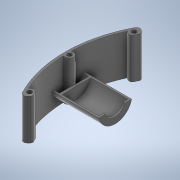
# Autodesk Inventor part: side_prot_cap
Saved by Autodesk Inventor 2020 (Build 240168000, 168)
## iProperties
Created: 2023-12-20
Part Number: side_prot_cap
Material: Пластик АБС
Document SubType Name: Modeling
Designer: denis
Density: 1.06 g/cm^3
Appearance: Гладкая — черная
Author: denis
## iProperties of the stored document _3DПЕЧАТЬ.ipt
Created: 2024-05-20
Part Number: _3DПЕЧАТЬ
Material: Типовые
Document SubType Name: Modeling
Designer: 4s
Density: 1 g/cm^3
Appearance: По умолчанию
Author: 4s
Autodesk Inventor part; units mm, degrees
(part 1 of 3)
ref_plane "XZ Plane" through (0, 0, 0) normal (0, 1, 0) x (-1, 0, 0)
sketch "Эскиз1" plane through (0, 0, 0) normal (0, 1, 0) x (-1, 0, 0)
  arc A0 (93.0503, -48.6481) -> (93.0503, 48.6481) centre (0, 0) ccw
  line L0 (0, 0) -> (0, -105) construction
  line L1 (0, 0) -> (105, 0) construction
  line L2 (0, 0) -> (74.2462, -74.2462) construction
  line L3 (0, 0) -> (105, 0) construction
  arc A1 (47.0668, -85.9577) -> (85.9577, -47.0668) centre (0, 0) ccw construction
  line L4 (0, 0) -> (-74.2462, -74.2462) construction
  line L5 (73.8927, -46.3155) -> (46.3155, -73.8927)
  line L6 (76.014, -34.2947) -> (34.2947, -76.014)
  circle A2 centre (37.8302, -79.5495) radius 1.6
  circle A3 centre (79.5495, -37.8302) radius 1.6
  line L7 (37.8302, -79.5495) -> (79.5495, -37.8302) construction
  line L8 (87.1795, -38.3892) -> (83.085, -34.2947)
  line L9 (38.3892, -87.1795) -> (34.2947, -83.085)
  line L10 (88.2704, -49.3795) -> (85.2064, -46.3155)
  line L11 (49.3795, -88.2704) -> (46.3155, -85.2064)
  arc A4 (74.2462, -74.2462) -> (91.1, -52.2091) centre (0, 0) ccw construction
  arc A5 (52.2091, -91.1) -> (74.2462, -74.2462) centre (0, 0) ccw construction
  arc A6 (48.6481, -93.0503) -> (49.3795, -88.2704) centre (47.2582, -90.3917) ccw
  arc A7 (88.2704, -49.3795) -> (93.0503, -48.6481) centre (90.3917, -47.2582) ccw
  arc A8 (46.3155, -73.8927) -> (46.3155, -85.2064) centre (51.9723, -79.5495) ccw
  arc A9 (85.2064, -46.3155) -> (73.8927, -46.3155) centre (79.5495, -51.9723) ccw
  arc A10 (34.2947, -76.014) -> (34.2947, -83.085) centre (37.8302, -79.5495) ccw
  arc A11 (83.085, -34.2947) -> (76.014, -34.2947) centre (79.5495, -37.8302) ccw
  arc A12 (40.4652, -89.2556) -> (47.0668, -85.9577) centre (0, 0) ccw construction
  arc A13 (85.9577, -47.0668) -> (89.2556, -40.4652) centre (0, 0) ccw construction
  arc A14 (90.4395, -37.7453) -> (90.4395, 37.7453) centre (0, 0) ccw
  arc A15 (87.1795, -38.3892) -> (90.4395, -37.7453) centre (88.5938, -36.975) ccw
  arc A16 (37.7453, -90.4395) -> (38.3892, -87.1795) centre (36.975, -88.5938) ccw
  arc A17 (38.3892, 87.1795) -> (37.7453, 90.4395) centre (36.975, 88.5938) ccw construction
  arc A18 (49.3795, 88.2704) -> (48.6481, 93.0503) centre (47.2582, 90.3917) ccw
  line L12 (49.3795, 88.2704) -> (46.3155, 85.2064)
  arc A19 (46.3155, 85.2064) -> (46.3155, 73.8927) centre (51.9723, 79.5495) ccw
  line L13 (38.3892, 87.1795) -> (34.2947, 83.085) construction
  arc A20 (34.2947, 83.085) -> (34.2947, 76.014) centre (37.8302, 79.5495) ccw construction
  line L14 (34.2947, 76.014) -> (76.014, 34.2947) construction
  line L15 (46.3155, 73.8927) -> (73.8927, 46.3155)
  arc A21 (76.014, 34.2947) -> (83.085, 34.2947) centre (79.5495, 37.8302) ccw
  circle A22 centre (37.8302, 79.5495) radius 1.6
  circle A23 centre (79.5495, 37.8302) radius 1.6
  line L16 (87.1795, 38.3892) -> (83.085, 34.2947)
  arc A24 (90.4395, 37.7453) -> (87.1795, 38.3892) centre (88.5938, 36.975) ccw
  arc A25 (93.0503, 48.6481) -> (88.2704, 49.3795) centre (90.3917, 47.2582) ccw
  line L17 (88.2704, 49.3795) -> (85.2064, 46.3155)
  arc A26 (73.8927, 46.3155) -> (85.2064, 46.3155) centre (79.5495, 51.9723) ccw
  arc A27 (-87.1795, 38.3892) -> (-90.4395, 37.7453) centre (-88.5938, 36.975) ccw
  arc A28 (-88.2704, 49.3795) -> (-93.0503, 48.6481) centre (-90.3917, 47.2582) ccw
  line L18 (-88.2704, 49.3795) -> (-85.2064, 46.3155)
  arc A29 (-85.2064, 46.3155) -> (-73.8927, 46.3155) centre (-79.5495, 51.9723) ccw
  line L19 (-87.1795, 38.3892) -> (-83.085, 34.2947)
  arc A30 (-83.085, 34.2947) -> (-76.014, 34.2947) centre (-79.5495, 37.8302) ccw
  line L20 (-76.014, 34.2947) -> (-34.2947, 76.014) construction
  line L21 (-73.8927, 46.3155) -> (-46.3155, 73.8927)
  arc A31 (-34.2947, 76.014) -> (-34.2947, 83.085) centre (-37.8302, 79.5495) ccw construction
  circle A32 centre (-79.5495, 37.8302) radius 1.6
  circle A33 centre (-37.8302, 79.5495) radius 1.6
  line L22 (-38.3892, 87.1795) -> (-34.2947, 83.085) construction
  arc A34 (-37.7453, 90.4395) -> (-38.3892, 87.1795) centre (-36.975, 88.5938) ccw construction
  arc A35 (-48.6481, 93.0503) -> (-49.3795, 88.2704) centre (-47.2582, 90.3917) ccw
  line L23 (-49.3795, 88.2704) -> (-46.3155, 85.2064)
  arc A36 (-46.3155, 73.8927) -> (-46.3155, 85.2064) centre (-51.9723, 79.5495) ccw
  arc A37 (-38.3892, -87.1795) -> (-37.7453, -90.4395) centre (-36.975, -88.5938) ccw
  arc A38 (-49.3795, -88.2704) -> (-48.6481, -93.0503) centre (-47.2582, -90.3917) ccw
  line L24 (-49.3795, -88.2704) -> (-46.3155, -85.2064)
  arc A39 (-46.3155, -85.2064) -> (-46.3155, -73.8927) centre (-51.9723, -79.5495) ccw
  line L25 (-38.3892, -87.1795) -> (-34.2947, -83.085)
  arc A40 (-34.2947, -83.085) -> (-34.2947, -76.014) centre (-37.8302, -79.5495) ccw
  line L26 (-34.2947, -76.014) -> (-76.014, -34.2947)
  line L27 (-46.3155, -73.8927) -> (-73.8927, -46.3155)
  arc A41 (-76.014, -34.2947) -> (-83.085, -34.2947) centre (-79.5495, -37.8302) ccw
  circle A42 centre (-37.8302, -79.5495) radius 1.6
  circle A43 centre (-79.5495, -37.8302) radius 1.6
  line L28 (-87.1795, -38.3892) -> (-83.085, -34.2947)
  arc A44 (-90.4395, -37.7453) -> (-87.1795, -38.3892) centre (-88.5938, -36.975) ccw
  arc A45 (-93.0503, -48.6481) -> (-88.2704, -49.3795) centre (-90.3917, -47.2582) ccw
  line L29 (-88.2704, -49.3795) -> (-85.2064, -46.3155)
  arc A46 (-73.8927, -46.3155) -> (-85.2064, -46.3155) centre (-79.5495, -51.9723) ccw
  arc A47 (0, 67.941) -> (23.7825, 76.5969) centre (0, 104.941) ccw construction
  arc A48 (-23.7825, 76.5969) -> (0, 67.941) centre (0, 104.941) ccw construction
  line L30 (-23.7825, 76.5969) -> (-29.1816, 81.127) construction
  arc A49 (-28.5452, 71.4571) -> (5.5413, 61.2914) centre (0, 104.941) ccw construction
  arc A50 (5.5413, 61.2914) -> (28.5452, 71.4571) centre (0, 104.941) ccw construction
  line L31 (23.7825, 76.5969) -> (26.8032, 79.1314) construction
  line L32 (-34.1491, 76.1596) -> (-28.5452, 71.4571) construction
  line L33 (31.2232, 73.7044) -> (28.5452, 71.4571) construction
  line L34 (26.8032, 79.1314) -> (23.7825, 76.5969) construction
  line L35 (30.7591, 79.5495) -> (31.4483, 78.8604) construction
  line L36 (31.2232, 73.7044) -> (28.5452, 71.4571) construction
  line L37 (-28.5452, 71.4571) -> (-34.1491, 76.1596) construction
  line L38 (-23.7825, 76.5969) -> (-29.1816, 81.127) construction
  line L39 (-29.1816, 81.127) -> (-34.1491, 76.1596) construction
  arc A51 (31.2232, 73.7044) -> (26.6462, 78.9996) centre (28.9734, 76.3855) ccw construction
  arc A52 (-26.6462, 78.9996) -> (-31.2232, 73.7044) centre (-28.9734, 76.3855) ccw construction
  arc A53 (-24.842, 61.8893) -> (-25.4187, 62.8242) centre (-28.1154, 60.5155) ccw
  line L40 (-24.842, 61.8893) -> (-23.8313, 59.4808)
  line L41 (-43.0355, 94.1655) -> (-18.3802, 65.3664)
  arc A54 (-0.6161, 59.3045) -> (0.6161, 59.3045) centre (0, 61.2072) ccw
  line L42 (-2.672, 59.9702) -> (-4.5, 60.5621) construction
  arc A55 (-2.5156, 60.0805) -> (-2.672, 59.9702) centre (0, 56.3493) ccw construction
  line L43 (-15.1585, 56.5907) -> (-21.0049, 57.3328)
  arc A56 (-14.5119, 56.4463) -> (-15.1585, 56.5907) centre (-15.6055, 53.069) ccw
  line L44 (-17.477, 64.7643) -> (-0.6161, 59.3045)
  line L45 (-14.5119, 56.4463) -> (-0.6161, 51.9466)
  arc A57 (44.0271, 95.3237) -> (43.577, 95.5303) centre (0, 0) ccw construction
  circle A58 centre (20.5578, 60.8546) radius 1.55
  arc A59 (-34.1909, 73.0707) -> (-37.1244, 73.1843) centre (-35.7102, 71.7701) ccw
  line L46 (-34.1909, 73.0707) -> (-27.0558, 64.7365) construction
  line L47 (-25.4187, 62.8242) -> (-34.1909, 73.0707)
  arc A60 (-23.8313, 59.4808) -> (-21.0049, 57.3328) centre (-20.5578, 60.8546) ccw
  arc A61 (-18.3802, 65.3664) -> (-17.477, 64.7643) centre (-16.8609, 66.6671) ccw
  circle A62 centre (-20.5578, 60.8546) radius 1.55
  arc A63 (15.1585, 56.5907) -> (14.5119, 56.4463) centre (15.6055, 53.069) ccw
  line L48 (15.1585, 56.5907) -> (21.0049, 57.3328)
  arc A64 (25.4187, 62.8242) -> (24.842, 61.8893) centre (28.1154, 60.5155) ccw
  line L49 (24.842, 61.8893) -> (23.8313, 59.4808)
  arc A65 (21.0049, 57.3328) -> (23.8313, 59.4808) centre (20.5578, 60.8546) ccw
  line L50 (25.4187, 62.8242) -> (34.1909, 73.0707)
  arc A66 (37.1244, 73.1843) -> (34.1909, 73.0707) centre (35.7102, 71.7701) ccw
  line L51 (14.5119, 56.4463) -> (0.6161, 51.9466)
  arc A67 (17.477, 64.7643) -> (18.3802, 65.3664) centre (16.8609, 66.6671) ccw
  line L52 (17.477, 64.7643) -> (0.6161, 59.3045)
  line L53 (-37.1244, 73.1843) -> (-76.014, 34.2947)
  line L54 (37.1244, 73.1843) -> (76.014, 34.2947)
  arc A68 (-45.42, 94.668) -> (-48.6481, 93.0503) centre (0, 0) ccw
  arc A69 (-43.0355, 94.1655) -> (-45.42, 94.668) centre (-44.5548, 92.8648) ccw
  arc A70 (-0.6161, 51.9466) -> (0.6161, 51.9466) centre (0, 53.8493) ccw
  arc A71 (-48.6481, 93.0503) -> (-93.0503, 48.6481) centre (0, 0) ccw construction
  line L55 (43.0355, 94.1655) -> (18.3802, 65.3664)
  arc A72 (48.6481, 93.0503) -> (45.42, 94.668) centre (0, 0) ccw
  arc A73 (45.42, 94.668) -> (43.0355, 94.1655) centre (44.5548, 92.8648) ccw
  arc A74 (93.0503, 48.6481) -> (-44.0271, 95.3237) centre (0, 0) ccw construction
  arc A75 (-93.0503, -48.6481) -> (-48.6481, -93.0503) centre (0, 0) ccw construction
  arc A76 (-93.0503, 48.6481) -> (-93.0503, -48.6481) centre (0, 0) ccw
  arc A77 (-90.4395, -37.7453) -> (-37.7453, -90.4395) centre (0, 0) ccw construction
  arc A78 (-90.4395, 37.7453) -> (-90.4395, -37.7453) centre (0, 0) ccw
  arc A79 (90.4395, 37.7453) -> (-90.4395, 37.7453) centre (0, 0) ccw construction
  arc A80 (-37.7453, -90.4395) -> (37.7453, -90.4395) centre (0, 0) ccw
  arc A81 (-48.6481, -93.0503) -> (48.6481, -93.0503) centre (0, 0) ccw
  circle A82 centre (0, 55.5993) radius 1.75
  point P0 (60.1041, -60.1041)
  point P1 (55.1543, -55.1543)
  point P2 (78.1353, -39.2444)
  point P3 (39.2444, -78.1353)
  point P4 (52.2091, 91.1)
  point P5 (39.2444, 78.1353)
  point P6 (47.0668, 85.9577)
  point P7 (55.1543, 55.1543)
  point P8 (60.1041, 60.1041)
  point P9 (91.1, 52.2091)
  point P10 (78.1353, 39.2444)
  point P11 (85.9577, 47.0668)
  point P12 (-91.1, 52.2091)
  point P13 (-78.1353, 39.2444)
  point P14 (-85.9577, 47.0668)
  point P15 (-55.1543, 55.1543)
  point P16 (-60.1041, 60.1041)
  point P17 (-52.2091, 91.1)
  point P18 (-39.2444, 78.1353)
  point P19 (-47.0668, 85.9577)
  point P20 (-52.2091, -91.1)
  point P21 (-39.2444, -78.1353)
  point P22 (-47.0668, -85.9577)
  point P23 (-55.1543, -55.1543)
  point P24 (-60.1041, -60.1041)
  point P25 (-91.1, -52.2091)
  point P26 (-78.1353, -39.2444)
  point P27 (-85.9577, -47.0668)
  point P28 (-28.5452, 71.4571)
  point P29 (-39.283, 89.7822)
  point P30 (0, 95.3237)
  point P31 (0, 66.2072)
  point P32 (-44.0271, 95.3237)
  point P33 (0, 59.2072)
  point P34 (44.5548, 92.8648)
  point P35 (-42.4264, 67.8823)
  point P36 (-22.7059, 58.0282)
  point P37 (-21.4957, 59.6205)
  dimension "d1" = 45
  dimension "d3" = 7
  dimension "d5" = 20
  dimension "d9" = 7
  dimension "d10" = 3.2
  dimension "d14" = 59
  dimension "d15" = 83
  dimension "d17" = 69
  dimension "d19" = 55
  dimension "d20" = 3
  dimension "d21" = 8
  dimension "d22" = 5
  dimension "d23" = 2
  dimension "d26" = 360
  dimension "d39" = 7
  dimension "d44" = 120
  dimension "d45" = 3.55
  dimension "d46" = 2
  dimension "d47" = 2.6119
  dimension "d48" = 2
  dimension "d49" = 105
  dimension "d50" = 2
  dimension "d54" = 3.5
  dimension "d55" = 2
  constraints: 165 point on circle, 112 end point, 83 centre point, 38 point on line, 27 tangent, 23 symmetric about line, 8 midpoint, 6 equal radius, 4 coincident, 4 collinear, 4 parallel, 3 horizontal, 2 vertical, 1 equal length, 1 perpendicular, 234 other
  measures "d1" angle of L2 L3
  measures "d3" radial gap between concentric circles of A0 A1
  measures "d5" distance from line of L5 L2.end
  measures "d9" distance between parallel lines of L5 L6
  measures "d10" diameter of A2
  measures "d14" distance of L7.end L7.start
  measures "d15" distance from line of point (0, 0) L7
  measures "d17" distance between parallel lines of L8 L9
  measures "d19" distance between parallel lines of L11 L10
  measures "d20" radius of A6
  measures "d21" radius of A8
  measures "d22" radius of A10
  measures "d23" radius of A15
  measures "d39" distance of point (0, 66.207) point (0, 59.207)
  measures "d44" angle of L40 L43
  measures "d45" radius of A53
  measures "d46" distance of point (-22.706, 58.028) point (-21.496, 59.621)
  measures "d47" distance of L40.start L40.end
  measures "d48" radius of A69
  measures "d49" radius of A68
  measures "d50" radius of A70
  measures "d54" diameter of A82
extrude "outer" add sketch "Эскиз1" along normal blind 2 contours A7 L10 A9 L5 A8 L11 A6 A81 A38 L24 A39 L27 A46 L29 A45 A76 A28 L18 A29 L21 A36 L23 A35 A68 A69 L41 A61 L44 A54 L52 A67 L55 A73 A72 A18 L12 A19 L15 A26 L17 A25 A0 | A82
sketch "Эскиз2" plane through (0, 2, 0) normal (0, 1, 0) x (1, 0, 0)
  arc A0 (-46.3155, -85.2064) -> (-46.3155, -73.8927) centre (-51.9723, -79.5495) ccw construction
  line L0 (-46.3155, -85.2064) -> (-49.3795, -88.2704) construction
  arc A1 (-49.3795, -88.2704) -> (-48.6481, -93.0503) centre (-47.2582, -90.3917) ccw construction
  arc A2 (-48.6481, -93.0503) -> (-45.42, -94.668) centre (0, 0) ccw construction
  arc A3 (-45.42, -94.668) -> (-43.0355, -94.1655) centre (-44.5548, -92.8648) ccw construction
  line L1 (-43.0355, -94.1655) -> (-18.3802, -65.3664) construction
  arc A4 (-17.477, -64.7643) -> (-18.3802, -65.3664) centre (-16.8609, -66.6671) ccw construction
  line L2 (-17.477, -64.7643) -> (-0.6161, -59.3045) construction
  arc A5 (0.6161, -59.3045) -> (-0.6161, -59.3045) centre (0, -61.2072) ccw construction
  line L3 (0.6161, -59.3045) -> (17.477, -64.7643) construction
  arc A6 (18.3802, -65.3664) -> (17.477, -64.7643) centre (16.8609, -66.6671) ccw construction
  line L4 (18.3802, -65.3664) -> (43.0355, -94.1655) construction
  arc A7 (43.0355, -94.1655) -> (45.42, -94.668) centre (44.5548, -92.8648) ccw construction
  arc A8 (45.42, -94.668) -> (48.6481, -93.0503) centre (0, 0) ccw construction
  arc A9 (48.6481, -93.0503) -> (49.3795, -88.2704) centre (47.2582, -90.3917) ccw construction
  line L5 (49.3795, -88.2704) -> (46.3155, -85.2064) construction
  arc A10 (46.3155, -73.8927) -> (46.3155, -85.2064) centre (51.9723, -79.5495) ccw construction
  line L6 (46.3155, -73.8927) -> (73.8927, -46.3155) construction
  arc A11 (85.2064, -46.3155) -> (73.8927, -46.3155) centre (79.5495, -51.9723) ccw construction
  line L7 (85.2064, -46.3155) -> (88.2704, -49.3795) construction
  arc A12 (88.2704, -49.3795) -> (93.0503, -48.6481) centre (90.3917, -47.2582) ccw construction
  arc A13 (93.0503, -48.6481) -> (93.0503, 48.6481) centre (0, 0) ccw construction
  arc A14 (93.0503, 48.6481) -> (88.2704, 49.3795) centre (90.3917, 47.2582) ccw construction
  line L8 (88.2704, 49.3795) -> (85.2064, 46.3155) construction
  arc A15 (73.8927, 46.3155) -> (85.2064, 46.3155) centre (79.5495, 51.9723) ccw construction
  line L9 (73.8927, 46.3155) -> (46.3155, 73.8927) construction
  arc A16 (46.3155, 85.2064) -> (46.3155, 73.8927) centre (51.9723, 79.5495) ccw construction
  line L10 (46.3155, 85.2064) -> (49.3795, 88.2704) construction
  arc A17 (49.3795, 88.2704) -> (48.6481, 93.0503) centre (47.2582, 90.3917) ccw construction
  arc A18 (48.6481, 93.0503) -> (-48.6481, 93.0503) centre (0, 0) ccw construction
  arc A19 (-48.6481, 93.0503) -> (-49.3795, 88.2704) centre (-47.2582, 90.3917) ccw construction
  line L11 (-49.3795, 88.2704) -> (-46.3155, 85.2064) construction
  arc A20 (-46.3155, 73.8927) -> (-46.3155, 85.2064) centre (-51.9723, 79.5495) ccw construction
  line L12 (-46.3155, 73.8927) -> (-73.8927, 46.3155) construction
  arc A21 (-85.2064, 46.3155) -> (-73.8927, 46.3155) centre (-79.5495, 51.9723) ccw construction
  line L13 (-85.2064, 46.3155) -> (-88.2704, 49.3795) construction
  arc A22 (-88.2704, 49.3795) -> (-93.0503, 48.6481) centre (-90.3917, 47.2582) ccw construction
  arc A23 (-93.0503, 48.6481) -> (-93.0503, -48.6481) centre (0, 0) ccw construction
  arc A24 (-93.0503, -48.6481) -> (-88.2704, -49.3795) centre (-90.3917, -47.2582) ccw construction
  line L14 (-88.2704, -49.3795) -> (-85.2064, -46.3155) construction
  arc A25 (-73.8927, -46.3155) -> (-85.2064, -46.3155) centre (-79.5495, -51.9723) ccw construction
  line L15 (-73.8927, -46.3155) -> (-46.3155, -73.8927) construction
  circle A26 centre (-37.8302, 79.5495) radius 1.6 construction
  circle A27 centre (-79.5495, 37.8302) radius 1.6 construction
  circle A28 centre (-79.5495, -37.8302) radius 1.6 construction
  circle A29 centre (79.5495, -37.8302) radius 1.6 construction
  circle A30 centre (37.8302, 79.5495) radius 1.6 construction
  circle A31 centre (79.5495, 37.8302) radius 1.6 construction
  circle A32 centre (-20.5578, -60.8546) radius 1.55 construction
  circle A33 centre (20.5578, -60.8546) radius 1.55 construction
  circle A34 centre (37.8302, -79.5495) radius 1.6 construction
  circle A35 centre (-37.8302, -79.5495) radius 1.6 construction
  line L16 (-83.085, -34.2947) -> (-87.1795, -38.3892) construction
  arc A36 (-90.4395, -37.7453) -> (-87.1795, -38.3892) centre (-88.5938, -36.975) ccw construction
  arc A37 (-90.4395, 37.7453) -> (-90.4395, -37.7453) centre (0, 0) ccw construction
  arc A38 (-87.1795, 38.3892) -> (-90.4395, 37.7453) centre (-88.5938, 36.975) ccw construction
  line L17 (-87.1795, 38.3892) -> (-83.085, 34.2947) construction
  arc A39 (-83.085, 34.2947) -> (-76.014, 34.2947) centre (-79.5495, 37.8302) ccw construction
  line L18 (-76.014, 34.2947) -> (-34.2947, 76.014) construction
  arc A40 (-34.2947, 76.014) -> (-34.2947, 83.085) centre (-37.8302, 79.5495) ccw construction
  line L19 (-34.2947, 83.085) -> (-38.3892, 87.1795) construction
  arc A41 (-37.7453, 90.4395) -> (-38.3892, 87.1795) centre (-36.975, 88.5938) ccw construction
  arc A42 (37.7453, 90.4395) -> (-37.7453, 90.4395) centre (0, 0) ccw construction
  arc A43 (38.3892, 87.1795) -> (37.7453, 90.4395) centre (36.975, 88.5938) ccw construction
  line L20 (38.3892, 87.1795) -> (34.2947, 83.085) construction
  arc A44 (34.2947, 83.085) -> (34.2947, 76.014) centre (37.8302, 79.5495) ccw construction
  line L21 (34.2947, 76.014) -> (76.014, 34.2947) construction
  arc A45 (76.014, 34.2947) -> (83.085, 34.2947) centre (79.5495, 37.8302) ccw construction
  line L22 (83.085, 34.2947) -> (87.1795, 38.3892) construction
  arc A46 (90.4395, 37.7453) -> (87.1795, 38.3892) centre (88.5938, 36.975) ccw construction
  arc A47 (90.4395, -37.7453) -> (90.4395, 37.7453) centre (0, 0) ccw construction
  arc A48 (87.1795, -38.3892) -> (90.4395, -37.7453) centre (88.5938, -36.975) ccw construction
  line L23 (87.1795, -38.3892) -> (83.085, -34.2947) construction
  arc A49 (83.085, -34.2947) -> (76.014, -34.2947) centre (79.5495, -37.8302) ccw construction
  line L24 (76.014, -34.2947) -> (37.1244, -73.1843) construction
  arc A50 (34.1909, -73.0707) -> (37.1244, -73.1843) centre (35.7102, -71.7701) ccw construction
  line L25 (34.1909, -73.0707) -> (25.4187, -62.8242) construction
  arc A51 (24.842, -61.8893) -> (25.4187, -62.8242) centre (28.1154, -60.5155) ccw construction
  line L26 (24.842, -61.8893) -> (23.8313, -59.4808) construction
  arc A52 (23.8313, -59.4808) -> (21.0049, -57.3328) centre (20.5578, -60.8546) ccw construction
  line L27 (21.0049, -57.3328) -> (15.1585, -56.5907) construction
  arc A53 (14.5119, -56.4463) -> (15.1585, -56.5907) centre (15.6055, -53.069) ccw construction
  line L28 (14.5119, -56.4463) -> (0.6161, -51.9466) construction
  arc A54 (0.6161, -51.9466) -> (-0.6161, -51.9466) centre (0, -53.8493) ccw construction
  line L29 (-0.6161, -51.9466) -> (-14.5119, -56.4463) construction
  arc A55 (-15.1585, -56.5907) -> (-14.5119, -56.4463) centre (-15.6055, -53.069) ccw construction
  line L30 (-15.1585, -56.5907) -> (-21.0049, -57.3328) construction
  arc A56 (-21.0049, -57.3328) -> (-23.8313, -59.4808) centre (-20.5578, -60.8546) ccw construction
  line L31 (-23.8313, -59.4808) -> (-24.842, -61.8893) construction
  arc A57 (-25.4187, -62.8242) -> (-24.842, -61.8893) centre (-28.1154, -60.5155) ccw construction
  line L32 (-25.4187, -62.8242) -> (-34.1909, -73.0707) construction
  arc A58 (-37.1244, -73.1843) -> (-34.1909, -73.0707) centre (-35.7102, -71.7701) ccw construction
  line L33 (-37.1244, -73.1843) -> (-76.014, -34.2947) construction
  arc A59 (-76.014, -34.2947) -> (-83.085, -34.2947) centre (-79.5495, -37.8302) ccw construction
  line L34 (0, 0) -> (-74.2462, 74.2462) construction
  line L35 (0, 0) -> (-105, 0) construction
  line L36 (0, 0) -> (0, 105) construction
  line L37 (0, 0) -> (74.2462, 74.2462) construction
  line L38 (-46.669, 63.6396) -> (-26.8701, 43.8406)
  line L39 (-63.6396, 46.669) -> (-43.8406, 26.8701)
  line L40 (-67.8823, 42.4264) -> (-43.1335, 17.6777) construction
  line L41 (-41.0122, 26.8701) -> (-26.8701, 41.0122)
  line L42 (-43.1347, 17.6765) -> (-17.6777, 43.1335) construction
  circle A60 centre (-21.9203, 43.1335) radius 1.6
  circle A61 centre (-43.1335, 21.9203) radius 1.6
  line L43 (-33.9411, 33.9411) -> (-30.4056, 30.4056) construction
  arc A62 (-26.8701, 41.0122) -> (-26.8701, 43.8406) centre (-28.2843, 42.4264) ccw
  arc A63 (-43.8406, 26.8701) -> (-41.0122, 26.8701) centre (-42.4264, 28.2843) ccw
  line L44 (-67.8823, 42.4264) -> (-42.4264, 67.8823)
  line L45 (-43.1335, 21.9203) -> (-21.9203, 43.1335) construction
  line L46 (-63.6396, -46.669) -> (-43.8406, -26.8701)
  line L47 (-42.4264, -67.8823) -> (-67.8823, -42.4264)
  line L48 (-46.669, -63.6396) -> (-26.8701, -43.8406)
  line L49 (-26.8701, -41.0122) -> (-41.0122, -26.8701)
  arc A64 (-41.0122, -26.8701) -> (-43.8406, -26.8701) centre (-42.4264, -28.2843) ccw
  circle A65 centre (-43.1335, -21.9203) radius 1.6
  circle A66 centre (-21.9203, -43.1335) radius 1.6
  arc A67 (-26.8701, -43.8406) -> (-26.8701, -41.0122) centre (-28.2843, -42.4264) ccw
  line L50 (46.669, -63.6396) -> (26.8701, -43.8406)
  line L51 (67.8823, -42.4264) -> (42.4264, -67.8823)
  line L52 (63.6396, -46.669) -> (43.8406, -26.8701)
  line L53 (41.0122, -26.8701) -> (26.8701, -41.0122)
  arc A68 (26.8701, -41.0122) -> (26.8701, -43.8406) centre (28.2843, -42.4264) ccw
  circle A69 centre (21.9203, -43.1335) radius 1.6
  circle A70 centre (43.1335, -21.9203) radius 1.6
  arc A71 (43.8406, -26.8701) -> (41.0122, -26.8701) centre (42.4264, -28.2843) ccw
  line L54 (63.6396, 46.669) -> (43.8406, 26.8701)
  line L55 (42.4264, 67.8823) -> (67.8823, 42.4264)
  line L56 (46.669, 63.6396) -> (26.8701, 43.8406)
  line L57 (26.8701, 41.0122) -> (41.0122, 26.8701)
  arc A72 (41.0122, 26.8701) -> (43.8406, 26.8701) centre (42.4264, 28.2843) ccw
  circle A73 centre (43.1335, 21.9203) radius 1.6
  circle A74 centre (21.9203, 43.1335) radius 1.6
  arc A75 (26.8701, 43.8406) -> (26.8701, 41.0122) centre (28.2843, 42.4264) ccw
  line L58 (-21.9203, 43.1335) -> (21.9203, 43.1335) construction
  line L59 (-20.6777, 40.1335) -> (20.6777, 40.1335) construction
  line L60 (-20.6777, 46.1335) -> (20.6777, 46.1335) construction
  line L61 (42.4264, 67.8823) -> (14.2253, 39.6811) construction
  line L62 (67.8823, 42.4264) -> (40.3188, 14.8629) construction
  line L63 (43.1347, 17.6765) -> (16.6158, 44.1954) construction
  arc A76 (-21.6698, 47.1257) -> (-21.6698, 39.1414) centre (-21.9203, 43.1335) ccw construction
  line L64 (-42.4264, 67.8823) -> (-21.6698, 47.1257)
  arc A77 (-19.2746, 46.1335) -> (-21.6698, 47.1257) centre (-21.9203, 43.1335) ccw
  arc A78 (-21.6698, 39.1414) -> (-19.2746, 40.1335) centre (-21.9203, 43.1335) ccw
  arc A79 (-19.2746, 40.1335) -> (-19.2746, 46.1335) centre (-21.9203, 43.1335) ccw construction
  line L65 (-21.6698, 47.1257) -> (-17.6777, 43.1335) construction
  line L66 (-19.2746, 46.1335) -> (0, 46.1335)
  line L67 (-30.4056, 30.4056) -> (-21.6698, 39.1414)
  line L68 (-67.8823, 42.4264) -> (-47.1257, 21.6698)
  arc A80 (-47.1257, 21.6698) -> (-46.1335, 19.2746) centre (-43.1335, 21.9203) ccw
  arc A81 (-40.1335, 19.2746) -> (-39.1414, 21.6698) centre (-43.1335, 21.9203) ccw
  line L69 (-46.1335, 19.2746) -> (-46.1335, 0)
  line L70 (-30.4056, 30.4056) -> (-39.1414, 21.6698)
  line L71 (-19.2746, 40.1335) -> (0, 40.1335)
  line L72 (-40.1335, 19.2746) -> (-40.1335, 0)
  line L73 (-40.1335, -19.2746) -> (-40.1335, 0)
  line L74 (-46.1335, -19.2746) -> (-46.1335, 0)
  arc A82 (-46.1335, -19.2746) -> (-47.1257, -21.6698) centre (-43.1335, -21.9203) ccw
  line L75 (-67.8823, -42.4264) -> (-47.1257, -21.6698)
  arc A83 (-39.1414, -21.6698) -> (-40.1335, -19.2746) centre (-43.1335, -21.9203) ccw
  line L76 (-30.4056, -30.4056) -> (-39.1414, -21.6698)
  line L77 (-30.4056, -30.4056) -> (-21.6698, -39.1414)
  arc A84 (-19.2746, -40.1335) -> (-21.6698, -39.1414) centre (-21.9203, -43.1335) ccw
  line L78 (-19.2746, -40.1335) -> (0, -40.1335)
  line L79 (-19.2746, -46.1335) -> (0, -46.1335)
  arc A85 (-21.6698, -47.1257) -> (-19.2746, -46.1335) centre (-21.9203, -43.1335) ccw
  line L80 (-42.4264, -67.8823) -> (-21.6698, -47.1257)
  line L81 (19.2746, -40.1335) -> (0, -40.1335)
  line L82 (19.2746, -46.1335) -> (0, -46.1335)
  arc A86 (19.2746, -46.1335) -> (21.6698, -47.1257) centre (21.9203, -43.1335) ccw
  line L83 (42.4264, -67.8823) -> (21.6698, -47.1257)
  arc A87 (21.6698, -39.1414) -> (19.2746, -40.1335) centre (21.9203, -43.1335) ccw
  line L84 (30.4056, -30.4056) -> (21.6698, -39.1414)
  line L85 (30.4056, -30.4056) -> (39.1414, -21.6698)
  arc A88 (40.1335, -19.2746) -> (39.1414, -21.6698) centre (43.1335, -21.9203) ccw
  line L86 (40.1335, -19.2746) -> (40.1335, 0)
  line L87 (46.1335, -19.2746) -> (46.1335, 0)
  arc A89 (47.1257, -21.6698) -> (46.1335, -19.2746) centre (43.1335, -21.9203) ccw
  line L88 (67.8823, -42.4264) -> (47.1257, -21.6698)
  line L89 (40.1335, 19.2746) -> (40.1335, 0)
  line L90 (46.1335, 19.2746) -> (46.1335, 0)
  arc A90 (46.1335, 19.2746) -> (47.1257, 21.6698) centre (43.1335, 21.9203) ccw
  line L91 (67.8823, 42.4264) -> (47.1257, 21.6698)
  arc A91 (39.1414, 21.6698) -> (40.1335, 19.2746) centre (43.1335, 21.9203) ccw
  line L92 (30.4056, 30.4056) -> (39.1414, 21.6698)
  line L93 (30.4056, 30.4056) -> (21.6698, 39.1414)
  arc A92 (19.2746, 40.1335) -> (21.6698, 39.1414) centre (21.9203, 43.1335) ccw
  line L94 (19.2746, 40.1335) -> (0, 40.1335)
  line L95 (19.2746, 46.1335) -> (0, 46.1335)
  arc A93 (21.6698, 47.1257) -> (19.2746, 46.1335) centre (21.9203, 43.1335) ccw
  line L96 (42.4264, 67.8823) -> (21.6698, 47.1257)
  point P0 (-25.4558, 42.4264)
  point P1 (-32.1734, 32.1734)
  point P2 (-42.4264, -25.4558)
  point P3 (-33.9411, -33.9411)
  point P4 (25.4558, -42.4264)
  point P5 (33.9411, -33.9411)
  point P6 (42.4264, 25.4558)
  point P7 (33.9411, 33.9411)
  point P8 (-46.1335, -20.6777)
  point P9 (20.6777, -46.1335)
  point P10 (46.1335, 20.6777)
  point P11 (0, 46.1335)
  point P12 (-46.1335, 0)
  point P13 (0, -46.1335)
  point P14 (46.1335, 0)
  point P15 (0, 40.1335)
  point P16 (40.1335, 0)
  point P17 (0, -40.1335)
  point P18 (-40.1335, 0)
  dimension "d58" = 12
  dimension "d59" = 30
  dimension "d60" = 5
  dimension "d61" = 3.2
  dimension "d62" = 30
  dimension "d63" = 2
  dimension "d64" = 2
  dimension "d65" = 3
  dimension "d68" = 360
  dimension "d70" = 6
  dimension "d71" = 8
  dimension "d74" = 360
  constraints: 118 end point, 52 point on circle, 34 centre point, 28 point on line, 8 symmetric about line, 5 parallel, 4 midpoint, 4 tangent, 1 coincident, 1 collinear, 1 horizontal, 1 perpendicular, 216 other
  measures "d58" distance between parallel lines of L34 L38
  measures "d59" distance between parallel lines of L18 L41
  measures "d60" distance between parallel lines of L41 L42
  measures "d61" diameter of A60
  measures "d62" distance of L45.start L45.end
  measures "d63" radius of A62
  measures "d64" radius of A63
  measures "d65" distance between parallel lines of L42 L45
  measures "d70" distance between parallel lines of L59 L60
  measures "d71" diameter of A76
extrude "inner" add sketch "Эскиз2" against normal blind 2 contours L44 L64 A77 L66 L95 A93 L96 L55 L56 A75 L57 A72 L54 L91 A90 L90 L87 A89 L88 L51 L52 A71 L53 A68 L50 L83 A86 L82 L79 A85 L80 L47 L48 A67 L49 A64 L46 L75 A82 L74 L69 A80 L68 L39 A63 L41 A62 L38
sketch "Эскиз3" plane through (0, 2, 0) normal (0, 1, 0) x (1, 0, 0)
  line L0 (-40.1335, -19.2746) -> (-40.1335, 19.2746) construction
  line L1 (-67.8823, -42.4264) -> (-76.014, -34.2947) construction
  arc A0 (-76.014, -34.2947) -> (-83.085, -34.2947) centre (-79.5495, -37.8302) ccw construction
  line L2 (-83.085, -34.2947) -> (-87.1795, -38.3892) construction
  arc A1 (-90.4395, -37.7453) -> (-87.1795, -38.3892) centre (-88.5938, -36.975) ccw construction
  arc A2 (-90.4395, 37.7453) -> (-90.4395, -37.7453) centre (0, 0) ccw construction
  arc A3 (-87.1795, 38.3892) -> (-90.4395, 37.7453) centre (-88.5938, 36.975) ccw construction
  line L3 (-87.1795, 38.3892) -> (-83.085, 34.2947) construction
  arc A4 (-83.085, 34.2947) -> (-76.014, 34.2947) centre (-79.5495, 37.8302) ccw construction
  line L4 (-76.014, 34.2947) -> (-67.8823, 42.4264) construction
  line L5 (-67.8823, 42.4264) -> (-47.1257, 21.6698) construction
  arc A5 (-47.1257, 21.6698) -> (-46.1335, 19.2746) centre (-43.1335, 21.9203) ccw construction
  line L6 (-46.1335, 19.2746) -> (-46.1335, -19.2746) construction
  arc A6 (-46.1335, -19.2746) -> (-47.1257, -21.6698) centre (-43.1335, -21.9203) ccw construction
  line L7 (-47.1257, -21.6698) -> (-67.8823, -42.4264) construction
  line L8 (-63.6396, -46.669) -> (-43.8406, -26.8701) construction
  arc A7 (-41.0122, -26.8701) -> (-43.8406, -26.8701) centre (-42.4264, -28.2843) ccw construction
  line L9 (-41.0122, -26.8701) -> (-26.8701, -41.0122) construction
  arc A8 (-26.8701, -43.8406) -> (-26.8701, -41.0122) centre (-28.2843, -42.4264) ccw construction
  line L10 (-26.8701, -43.8406) -> (-46.669, -63.6396) construction
  line L11 (-46.669, -63.6396) -> (-63.6396, -46.669) construction
  line L12 (-42.4264, -67.8823) -> (-21.6698, -47.1257) construction
  arc A9 (-21.6698, -47.1257) -> (-19.2746, -46.1335) centre (-21.9203, -43.1335) ccw construction
  line L13 (-19.2746, -46.1335) -> (19.2746, -46.1335) construction
  arc A10 (19.2746, -46.1335) -> (21.6698, -47.1257) centre (21.9203, -43.1335) ccw construction
  line L14 (21.6698, -47.1257) -> (42.4264, -67.8823) construction
  line L15 (42.4264, -67.8823) -> (37.1244, -73.1843) construction
  arc A11 (34.1909, -73.0707) -> (37.1244, -73.1843) centre (35.7102, -71.7701) ccw construction
  line L16 (34.1909, -73.0707) -> (25.4187, -62.8242) construction
  arc A12 (24.842, -61.8893) -> (25.4187, -62.8242) centre (28.1154, -60.5155) ccw construction
  line L17 (24.842, -61.8893) -> (23.8313, -59.4808) construction
  arc A13 (23.8313, -59.4808) -> (21.0049, -57.3328) centre (20.5578, -60.8546) ccw construction
  line L18 (21.0049, -57.3328) -> (15.1585, -56.5907) construction
  arc A14 (14.5119, -56.4463) -> (15.1585, -56.5907) centre (15.6055, -53.069) ccw construction
  line L19 (14.5119, -56.4463) -> (0.6161, -51.9466) construction
  arc A15 (0.6161, -51.9466) -> (-0.6161, -51.9466) centre (0, -53.8493) ccw construction
  line L20 (-0.6161, -51.9466) -> (-14.5119, -56.4463) construction
  arc A16 (-15.1585, -56.5907) -> (-14.5119, -56.4463) centre (-15.6055, -53.069) ccw construction
  line L21 (-15.1585, -56.5907) -> (-21.0049, -57.3328) construction
  arc A17 (-21.0049, -57.3328) -> (-23.8313, -59.4808) centre (-20.5578, -60.8546) ccw construction
  line L22 (-23.8313, -59.4808) -> (-24.842, -61.8893) construction
  arc A18 (-25.4187, -62.8242) -> (-24.842, -61.8893) centre (-28.1154, -60.5155) ccw construction
  line L23 (-25.4187, -62.8242) -> (-34.1909, -73.0707) construction
  arc A19 (-37.1244, -73.1843) -> (-34.1909, -73.0707) centre (-35.7102, -71.7701) ccw construction
  line L24 (-37.1244, -73.1843) -> (-42.4264, -67.8823) construction
  line L25 (46.669, -63.6396) -> (26.8701, -43.8406) construction
  arc A20 (26.8701, -41.0122) -> (26.8701, -43.8406) centre (28.2843, -42.4264) ccw construction
  line L26 (26.8701, -41.0122) -> (41.0122, -26.8701) construction
  arc A21 (43.8406, -26.8701) -> (41.0122, -26.8701) centre (42.4264, -28.2843) ccw construction
  line L27 (43.8406, -26.8701) -> (63.6396, -46.669) construction
  line L28 (63.6396, -46.669) -> (46.669, -63.6396) construction
  line L29 (67.8823, -42.4264) -> (47.1257, -21.6698) construction
  arc A22 (47.1257, -21.6698) -> (46.1335, -19.2746) centre (43.1335, -21.9203) ccw construction
  line L30 (46.1335, -19.2746) -> (46.1335, 19.2746) construction
  arc A23 (46.1335, 19.2746) -> (47.1257, 21.6698) centre (43.1335, 21.9203) ccw construction
  line L31 (47.1257, 21.6698) -> (67.8823, 42.4264) construction
  line L32 (67.8823, 42.4264) -> (76.014, 34.2947) construction
  arc A24 (76.014, 34.2947) -> (83.085, 34.2947) centre (79.5495, 37.8302) ccw construction
  line L33 (83.085, 34.2947) -> (87.1795, 38.3892) construction
  arc A25 (90.4395, 37.7453) -> (87.1795, 38.3892) centre (88.5938, 36.975) ccw construction
  arc A26 (90.4395, -37.7453) -> (90.4395, 37.7453) centre (0, 0) ccw construction
  arc A27 (87.1795, -38.3892) -> (90.4395, -37.7453) centre (88.5938, -36.975) ccw construction
  line L34 (87.1795, -38.3892) -> (83.085, -34.2947) construction
  arc A28 (83.085, -34.2947) -> (76.014, -34.2947) centre (79.5495, -37.8302) ccw construction
  line L35 (76.014, -34.2947) -> (67.8823, -42.4264) construction
  line L36 (63.6396, 46.669) -> (43.8406, 26.8701) construction
  arc A29 (41.0122, 26.8701) -> (43.8406, 26.8701) centre (42.4264, 28.2843) ccw construction
  line L37 (41.0122, 26.8701) -> (26.8701, 41.0122) construction
  arc A30 (26.8701, 43.8406) -> (26.8701, 41.0122) centre (28.2843, 42.4264) ccw construction
  line L38 (26.8701, 43.8406) -> (46.669, 63.6396) construction
  line L39 (46.669, 63.6396) -> (63.6396, 46.669) construction
  line L40 (42.4264, 67.8823) -> (21.6698, 47.1257) construction
  arc A31 (21.6698, 47.1257) -> (19.2746, 46.1335) centre (21.9203, 43.1335) ccw construction
  line L41 (19.2746, 46.1335) -> (-19.2746, 46.1335) construction
  arc A32 (-19.2746, 46.1335) -> (-21.6698, 47.1257) centre (-21.9203, 43.1335) ccw construction
  line L42 (-21.6698, 47.1257) -> (-42.4264, 67.8823) construction
  line L43 (-42.4264, 67.8823) -> (-34.2947, 76.014) construction
  arc A33 (-34.2947, 76.014) -> (-34.2947, 83.085) centre (-37.8302, 79.5495) ccw construction
  line L44 (-34.2947, 83.085) -> (-38.3892, 87.1795) construction
  arc A34 (-37.7453, 90.4395) -> (-38.3892, 87.1795) centre (-36.975, 88.5938) ccw construction
  arc A35 (37.7453, 90.4395) -> (-37.7453, 90.4395) centre (0, 0) ccw construction
  arc A36 (38.3892, 87.1795) -> (37.7453, 90.4395) centre (36.975, 88.5938) ccw construction
  line L45 (38.3892, 87.1795) -> (34.2947, 83.085) construction
  arc A37 (34.2947, 83.085) -> (34.2947, 76.014) centre (37.8302, 79.5495) ccw construction
  line L46 (34.2947, 76.014) -> (42.4264, 67.8823) construction
  line L47 (-19.2746, 40.1335) -> (19.2746, 40.1335) construction
  arc A38 (19.2746, 40.1335) -> (21.6698, 39.1414) centre (21.9203, 43.1335) ccw construction
  line L48 (21.6698, 39.1414) -> (39.1414, 21.6698) construction
  arc A39 (39.1414, 21.6698) -> (40.1335, 19.2746) centre (43.1335, 21.9203) ccw construction
  line L49 (40.1335, 19.2746) -> (40.1335, -19.2746) construction
  arc A40 (40.1335, -19.2746) -> (39.1414, -21.6698) centre (43.1335, -21.9203) ccw construction
  line L50 (39.1414, -21.6698) -> (21.6698, -39.1414) construction
  arc A41 (21.6698, -39.1414) -> (19.2746, -40.1335) centre (21.9203, -43.1335) ccw construction
  line L51 (19.2746, -40.1335) -> (-19.2746, -40.1335) construction
  arc A42 (-19.2746, -40.1335) -> (-21.6698, -39.1414) centre (-21.9203, -43.1335) ccw construction
  line L52 (-21.6698, -39.1414) -> (-39.1414, -21.6698) construction
  arc A43 (-39.1414, -21.6698) -> (-40.1335, -19.2746) centre (-43.1335, -21.9203) ccw construction
  line L53 (-40.1335, -19.2746) -> (-40.1335, 19.2746) construction
  arc A44 (-40.1335, 19.2746) -> (-39.1414, 21.6698) centre (-43.1335, 21.9203) ccw construction
  line L54 (-39.1414, 21.6698) -> (-21.6698, 39.1414) construction
  arc A45 (-21.6698, 39.1414) -> (-19.2746, 40.1335) centre (-21.9203, 43.1335) ccw construction
  circle A46 centre (43.1335, 21.9203) radius 1.6 construction
  circle A47 centre (21.9203, -43.1335) radius 1.6 construction
  circle A48 centre (-21.9203, -43.1335) radius 1.6 construction
  circle A49 centre (-43.1335, -21.9203) radius 1.6 construction
  circle A50 centre (-43.1335, 21.9203) radius 1.6 construction
  circle A51 centre (-21.9203, 43.1335) radius 1.6 construction
  circle A52 centre (43.1335, -21.9203) radius 1.6 construction
  circle A53 centre (21.9203, 43.1335) radius 1.6 construction
  arc A54 (-88.2704, 49.3795) -> (-93.0503, 48.6481) centre (-90.3917, 47.2582) ccw construction
  arc A55 (-93.0503, 48.6481) -> (-93.0503, -48.6481) centre (0, 0) ccw construction
  arc A56 (-93.0503, -48.6481) -> (-88.2704, -49.3795) centre (-90.3917, -47.2582) ccw construction
  line L55 (-88.2704, -49.3795) -> (-85.2064, -46.3155) construction
  arc A57 (-73.8927, -46.3155) -> (-85.2064, -46.3155) centre (-79.5495, -51.9723) ccw construction
  line L56 (-73.8927, -46.3155) -> (-46.3155, -73.8927) construction
  arc A58 (-46.3155, -85.2064) -> (-46.3155, -73.8927) centre (-51.9723, -79.5495) ccw construction
  line L57 (-46.3155, -85.2064) -> (-49.3795, -88.2704) construction
  arc A59 (-49.3795, -88.2704) -> (-48.6481, -93.0503) centre (-47.2582, -90.3917) ccw construction
  arc A60 (-48.6481, -93.0503) -> (-45.42, -94.668) centre (0, 0) ccw construction
  arc A61 (-45.42, -94.668) -> (-43.0355, -94.1655) centre (-44.5548, -92.8648) ccw construction
  line L58 (-43.0355, -94.1655) -> (-18.3802, -65.3664) construction
  arc A62 (-17.477, -64.7643) -> (-18.3802, -65.3664) centre (-16.8609, -66.6671) ccw construction
  line L59 (-17.477, -64.7643) -> (-0.6161, -59.3045) construction
  arc A63 (0.6161, -59.3045) -> (-0.6161, -59.3045) centre (0, -61.2072) ccw construction
  line L60 (0.6161, -59.3045) -> (17.477, -64.7643) construction
  arc A64 (18.3802, -65.3664) -> (17.477, -64.7643) centre (16.8609, -66.6671) ccw construction
  line L61 (18.3802, -65.3664) -> (43.0355, -94.1655) construction
  arc A65 (43.0355, -94.1655) -> (45.42, -94.668) centre (44.5548, -92.8648) ccw construction
  arc A66 (45.42, -94.668) -> (48.6481, -93.0503) centre (0, 0) ccw construction
  arc A67 (48.6481, -93.0503) -> (49.3795, -88.2704) centre (47.2582, -90.3917) ccw construction
  line L62 (49.3795, -88.2704) -> (46.3155, -85.2064) construction
  arc A68 (46.3155, -73.8927) -> (46.3155, -85.2064) centre (51.9723, -79.5495) ccw construction
  line L63 (46.3155, -73.8927) -> (73.8927, -46.3155) construction
  arc A69 (85.2064, -46.3155) -> (73.8927, -46.3155) centre (79.5495, -51.9723) ccw construction
  line L64 (85.2064, -46.3155) -> (88.2704, -49.3795) construction
  arc A70 (88.2704, -49.3795) -> (93.0503, -48.6481) centre (90.3917, -47.2582) ccw construction
  arc A71 (93.0503, -48.6481) -> (93.0503, 48.6481) centre (0, 0) ccw construction
  arc A72 (93.0503, 48.6481) -> (88.2704, 49.3795) centre (90.3917, 47.2582) ccw construction
  line L65 (88.2704, 49.3795) -> (85.2064, 46.3155) construction
  arc A73 (73.8927, 46.3155) -> (85.2064, 46.3155) centre (79.5495, 51.9723) ccw construction
  line L66 (73.8927, 46.3155) -> (46.3155, 73.8927) construction
  arc A74 (46.3155, 85.2064) -> (46.3155, 73.8927) centre (51.9723, 79.5495) ccw construction
  line L67 (46.3155, 85.2064) -> (49.3795, 88.2704) construction
  arc A75 (49.3795, 88.2704) -> (48.6481, 93.0503) centre (47.2582, 90.3917) ccw construction
  arc A76 (48.6481, 93.0503) -> (-48.6481, 93.0503) centre (0, 0) ccw construction
  arc A77 (-48.6481, 93.0503) -> (-49.3795, 88.2704) centre (-47.2582, 90.3917) ccw construction
  line L68 (-49.3795, 88.2704) -> (-46.3155, 85.2064) construction
  arc A78 (-46.3155, 73.8927) -> (-46.3155, 85.2064) centre (-51.9723, 79.5495) ccw construction
  line L69 (-46.3155, 73.8927) -> (-73.8927, 46.3155) construction
  arc A79 (-85.2064, 46.3155) -> (-73.8927, 46.3155) centre (-79.5495, 51.9723) ccw construction
  line L70 (-85.2064, 46.3155) -> (-88.2704, 49.3795) construction
  circle A80 centre (-37.8302, 79.5495) radius 1.6 construction
  circle A81 centre (-79.5495, 37.8302) radius 1.6 construction
  circle A82 centre (-79.5495, -37.8302) radius 1.6 construction
  circle A83 centre (79.5495, -37.8302) radius 1.6 construction
  circle A84 centre (37.8302, 79.5495) radius 1.6 construction
  circle A85 centre (79.5495, 37.8302) radius 1.6 construction
  circle A86 centre (-20.5578, -60.8546) radius 1.55 construction
  circle A87 centre (20.5578, -60.8546) radius 1.55 construction
  circle A88 centre (37.8302, -79.5495) radius 1.6 construction
  circle A89 centre (-37.8302, -79.5495) radius 1.6 construction
  line L71 (-46.669, 63.6396) -> (-26.8701, 43.8406) construction
  arc A90 (-26.8701, 41.0122) -> (-26.8701, 43.8406) centre (-28.2843, 42.4264) ccw construction
  line L72 (-26.8701, 41.0122) -> (-41.0122, 26.8701) construction
  arc A91 (-43.8406, 26.8701) -> (-41.0122, 26.8701) centre (-42.4264, 28.2843) ccw construction
  line L73 (-43.8406, 26.8701) -> (-63.6396, 46.669) construction
  line L74 (-63.6396, 46.669) -> (-46.669, 63.6396) construction
  circle A92 centre (0, 0) radius 101 construction
  circle A93 centre (-101, 0) radius 1.9
  circle A94 centre (-101, 0) radius 4
  line L75 (0, 0) -> (0, 40.1335) construction
  line L76 (19.2746, 40.1335) -> (-19.2746, 40.1335) construction
  line L77 (0, 0) -> (-40.1335, 0) construction
  circle A95 centre (101, 0) radius 1.9
  circle A96 centre (101, 0) radius 4
  circle A97 centre (-90.3659, -45.1111) radius 2
  line L78 (-46.669, -63.6396) -> (-63.6396, -46.669) construction
  line L79 (-55.1543, -55.1543) -> (-33.9411, -33.9411) construction
  circle A98 centre (-45.1111, -90.3659) radius 2
  circle A99 centre (-90.3659, 45.1111) radius 2
  circle A100 centre (-45.1111, 90.3659) radius 2
  circle A101 centre (90.3659, -45.1111) radius 2
  circle A102 centre (45.1111, -90.3659) radius 2
  circle A103 centre (45.1111, 90.3659) radius 2
  circle A104 centre (90.3659, 45.1111) radius 2
  dimension "d78" = 202
  dimension "d79" = 3.8
  dimension "d80" = 8
  dimension "d81" = 4
  dimension "d84" = 64
  constraints: 13 centre point, 9 symmetric about line, 6 end point, 4 coincident, 4 midpoint, 2 point on circle, 9 other
  measures "d78" diameter of A92
  measures "d79" diameter of A93
  measures "d80" diameter of A94
  measures "d81" diameter of A97
  measures "d84" distance of A97.centre A98.centre
extrude "Выдавливание3" cut sketch "Эскиз3" against normal blind 10 contours A93 | A95 | A97 | A98 | A99 | A100 | A101 | A102 | A103 | A104
extrude "Выдавливание4" add sketch "Эскиз3" against normal blind 2 contours A94 | A96